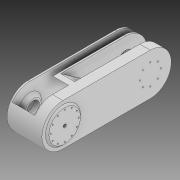
# Autodesk Inventor part: Link1
Saved by Autodesk Inventor 2020 (Build 240168000, 168)
## iProperties
Created: 2021-03-19
Part Number: Link1
Material: Generic
Document SubType Name: Modeling
Designer: DDeGo
Density: 1 g/cm^3
Appearance: Default
Author: DDeGo
Autodesk Inventor part; units mm, degrees
ref_plane "YZ Plane" through (0, 0, 0) normal (1, 0, 0) x (0, 1, 0)
ref_plane "XZ Plane" through (0, 0, 0) normal (0, 1, 0) x (-1, 0, 0)
ref_plane "XY Plane" through (0, 0, 0) normal (0, 0, 1) x (1, 0, 0)
sketch "Sketch1" plane through (0, 0, 0) normal (1, 0, 0) x (0, 1, 0)
  line L0 (0, 0) -> (0, -250) construction
  line L1 (-60, 0) -> (-60, -250)
  line L2 (60, -250) -> (60, 0)
  arc A0 (60, 0) -> (-60, 0) centre (0, 0) ccw
  arc A1 (-60, -250) -> (60, -250) centre (0, -250) ccw
  circle A2 centre (0, 0) radius 25 construction
  circle A3 centre (0, -250) radius 25
  point P0 (0, -125)
  dimension "d0" = 60
  dimension "d1" = 250
  dimension "d2" = 50
  constraints: 8 end point, 4 centre point, 4 point on circle, 4 tangent, 2 coincident, 1 equal radius, 1 midpoint, 1 parallel, 1 vertical
  measures "d0" radius of A0
  measures "d1" distance of L0.start L0.end
  measures "d2" diameter of A2
extrude "Extrusion1" add sketch "Sketch1" along normal blind 100
sketch "Sketch2" plane through (0, 60, 0) normal (0, 1, 0) x (1, 0, 0)
  line L0 (70, 185) -> (30, 185)
  line L1 (30, 185) -> (30, 315)
  line L2 (30, 315) -> (70, 315)
  line L3 (70, 315) -> (70, 185)
  line L4 (0, 250) -> (100, 250) construction
  line L5 (70, 185) -> (30, 315) construction
  line L6 (30, 185) -> (70, 315) construction
  line L7 (0, 310) -> (100, 310) construction
  line L8 (0, 250) -> (0, 310) projected
  line L9 (100, 250) -> (100, 310) projected
  point P0 (0, 0)
  point P1 (50, 250)
  dimension "d5" = 5
  dimension "d24" = 30
  dimension "d25" = 30
  constraints: 12 end point, 3 midpoint, 2 parallel, 1 horizontal, 1 perpendicular
  measures "d5" distance between parallel lines of L2 L7
  measures "d24" distance between parallel lines of L8 L1
  measures "d25" distance between parallel lines of L9 L3
extrude "Extrusion2" cut sketch "Sketch2" against normal through all
sketch "Sketch3" plane through (70, 60, -250) normal (-1, 0, 0) x (0, 0, 1)
  line L0 (0, 0) -> (65, 0) projected
  line L1 (65, 0) -> (186.3926, 0)
  line L2 (186.3926, 0) -> (65, -85)
  line L3 (65, 0) -> (65, -120) projected
  line L4 (65, -85) -> (65, 0)
  point P0 (250, -60)
  dimension "d10" = 85
  dimension "d13" = 55
  constraints: 6 end point, 1 horizontal, 1 perpendicular, 1 point on line
  measures "d10" distance of L0.end L2.end
  measures "d13" angle of L3 L2
extrude "Extrusion3" cut sketch "Sketch3" along normal up to surface (40 mm away)
sketch "Sketch4" plane through (100, 0, 0) normal (1, 0, 0) x (0, 0, -1)
  circle A0 centre (0, 0) radius 50
  dimension "d14" = 100
  constraints: 1 centre point, 1 coincident
  measures "d14" diameter of A0
extrude "Extrusion4" add sketch "Sketch4" along normal blind 5
sketch "Sketch5" plane through (105, 0, 0) normal (1, 0, 0) x (0, 0, -1)
  line L0 (0, 0) -> (40, 0) construction
  circle A0 centre (40, 0) radius 1.65
  dimension "d17" = 40
  dimension "d18" = 3.3
  constraints: 2 end point, 1 centre point, 1 coincident, 1 horizontal
  measures "d17" distance of L0.start L0.end
  measures "d18" diameter of A0
extrude "Extrusion5" cut sketch "Sketch5" against normal blind 15
pattern_circular "Circular Pattern1" count 12 over 360 about axis through (100, 0, 0) along (1, 0, 0) of "Extrusion5"
ref_plane "Work Plane1" through (5, 0, 0) normal (-1, 0, 0) x (0, 0, 1)
ref_plane "Work Plane2" through (25, 0, -250) normal (1, 0, 0) x (0, 0, -1)
sketch "Sketch7" plane through (5, 0, 0) normal (-1, 0, 0) x (0, 0, 1)
  arc A0 (0, -60) -> (0, 60) centre (0, 0) ccw projected
  line L0 (-250, 60) -> (0, 60) projected
  arc A1 (-250, 60) -> (-250, -60) centre (-250, 0) ccw projected
  line L1 (0, -60) -> (-250, -60) projected
  circle A2 centre (-250, 0) radius 25 construction
  arc A3 (0, -50) -> (50, 0) centre (0, 0) ccw
  line L2 (0, -50) -> (-250, -50)
  arc A4 (-250, 50) -> (-300, 0) centre (-250, 0) ccw construction
  line L3 (-250, 50) -> (0, 50) construction
  line L4 (50, 0) -> (50, 114.8918)
  line L5 (50, 114.8918) -> (-300, 114.8918)
  line L6 (-300, 114.8918) -> (-300, 0)
  arc A5 (50, 0) -> (0, 50) centre (0, 0) ccw construction
  arc A6 (-300, 0) -> (-250, -50) centre (-250, 0) ccw
  point P0 (-300, 33.1662)
  point P1 (50, 33.1662)
  dimension "d31" = 10
  dimension "d32" = 10
  dimension "d33" = 10
  constraints: 10 end point, 8 point on circle, 4 centre point, 2 vertical, 1 perpendicular
  measures "d31" distance between parallel lines of L1 L2
  measures "d32" radial gap between concentric circles of A0 A3
  measures "d33" radial gap between concentric circles of A1 A6
extrude "Extrusion6" cut sketch "Sketch7" against normal up to surface (20 mm away) contours L4 A3 L2 A6 L6 A1 L0 A0
sketch "Sketch8" plane through (25, 0, -300) normal (-1, 0, 0) x (0, 0, 1)
  circle A0 centre (50, 0) radius 25 projected
  line L0 (50, 60) -> (300, 60) projected
  arc A1 (50, 60) -> (0, 33.1662) centre (50, 0) ccw projected
  line L1 (0, 33.1662) -> (0, 0) projected
  arc A2 (0, 0) -> (50, -50) centre (50, 0) ccw projected
  line L2 (50, -50) -> (300, -50) projected
  arc A3 (300, -50) -> (350, 0) centre (300, 0) ccw projected
  line L3 (350, 0) -> (350, 33.1662) projected
  arc A4 (350, 33.1662) -> (300, 60) centre (300, 0) ccw projected
  line L4 (236.3926, 60) -> (115, -25) projected
  line L5 (115, -25) -> (236.3926, 60) projected
  line L6 (115, -25) -> (115, -60) projected
  line L7 (115, -25) -> (115, -60) projected
  line L8 (50, 60) -> (300, 60) projected
  line L9 (253.827, 60) -> (115, -37.2077)
  point P0 (115, -37.2077)
  point P1 (115, -50)
  dimension "d37" = 10
  constraints: 2 end point, 2 point on line, 1 parallel
  measures "d37" distance between parallel lines of L4 L9
extrude "Extrusion7" cut sketch "Sketch8" against normal up to surface (45 mm away) contours L0 A4 L3 A3 L2 L6 L9
sketch "Sketch9" plane through (0, 0, 0) normal (-1, 0, 0) x (0, 0, 1)
  circle A0 centre (0, 0) radius 17.6
  dimension "d40" = 35.2
  constraints: 1 centre point, 1 coincident
  measures "d40" diameter of A0
extrude "Extrusion8" cut sketch "Sketch9" against normal up to surface (5 mm away)
sketch "Sketch10" plane through (5, 0, 0) normal (1, 0, 0) x (0, 0, -1)
  circle A0 centre (0, 0) radius 17.6 projected
  circle A1 centre (0, 0) radius 22.6
  dimension "d43" = 5
  constraints: 1 centre point, 1 coincident
  measures "d43" radial gap between concentric circles of A1 A0
extrude "Extrusion9" add sketch "Sketch10" along normal blind 10
sketch "Sketch11" plane through (70, 0, -250) normal (-1, 0, 0) x (0, 0, 1)
  circle A0 centre (250, 0) radius 17.6 projected
  circle A1 centre (250, 0) radius 22.6
  dimension "d46" = 5
  constraints: 1 centre point, 1 coincident
  measures "d46" radial gap between concentric circles of A1 A0
extrude "Extrusion10" add sketch "Sketch11" along normal blind 10
fillet "Fillet1" radius 2 1 edges at (60, 0, -17.6)
sketch "Sketch12" plane through (105, 0, 0) normal (1, 0, 0) x (0, 0, -1)
  line L0 (4.792, 0) -> (2.396, -4.15)
  line L1 (2.396, -4.15) -> (-2.396, -4.15)
  line L2 (-2.396, -4.15) -> (-4.792, 0)
  line L3 (-4.792, 0) -> (-2.396, 4.15)
  line L4 (-2.396, 4.15) -> (2.396, 4.15)
  line L5 (2.396, 4.15) -> (4.792, 0)
  point P0 (0, 0)
  point P1 (0, 0)
  dimension "d50" = 8.3
  constraints: 12 end point, 1 coincident, 1 horizontal, 13 other
  measures "d50" distance between parallel lines of L1 L4
extrude "Extrusion11" cut sketch "Sketch12" against normal blind 6
sketch "Sketch13" plane through (99, 0, 0) normal (1, 0, 0) x (0, 0, -1)
  circle A0 centre (0, 0) radius 2.65
  dimension "d53" = 5.3
  constraints: 1 centre point, 1 coincident
  measures "d53" diameter of A0
extrude "Extrusion12" cut sketch "Sketch13" against normal blind 10
chamfer "Chamfer1" distance 10 angle 45 2 edges at (70, 0, -22.6) (5, 0, 22.6)
chamfer "Chamfer2" distance 5 angle 45 1 edges at (105, 0, 50)
sketch "Sketch14" plane through (70, 0, -250) normal (-1, 0, 0) x (0, 0, 1)
  circle A0 centre (0, 0) radius 25 projected
  circle A1 centre (0, 0) radius 47.55
  point P0 (250, 0)
  dimension "d62" = 95.1
  constraints: 1 centre point, 1 coincident
  measures "d62" diameter of A1
extrude "Extrusion13" cut sketch "Sketch14" against normal blind 10
sketch "Sketch15" plane through (80, 0, -250) normal (-1, 0, 0) x (0, 0, 1)
  circle A0 centre (0, 0) radius 25 projected
  circle A1 centre (0, 0) radius 44.55
  circle A2 centre (0, 0) radius 47.55 projected
  point P0 (250, 0)
  dimension "d65" = 3
  constraints: 1 centre point, 1 coincident
  measures "d65" radial gap between concentric circles of A2 A1
extrude "Extrusion14" cut sketch "Sketch15" against normal blind 0.5 contours A1
sketch "Sketch16" plane through (80.5, 0, -250) normal (-1, 0, 0) x (0, 0, 1)
  circle A0 centre (0, 0) radius 25 projected
  circle A1 centre (0, 0) radius 40
  point P0 (250, 0)
  dimension "d68" = 80
  constraints: 1 centre point, 1 coincident
  measures "d68" diameter of A1
extrude "Extrusion15" cut sketch "Sketch16" against normal blind 15.5
sketch "Sketch17" plane through (100, 0, 0) normal (1, 0, 0) x (0, 0, -1)
  circle A0 centre (250, 0) radius 25 construction
  circle A1 centre (250, 0) radius 30 construction
  circle A2 centre (250, 30) radius 1.6
  circle A3 centre (228.7868, 21.2132) radius 1.6
  circle A4 centre (220, 0) radius 1.6
  circle A5 centre (228.7868, -21.2132) radius 1.6
  circle A6 centre (250, -30) radius 1.6
  circle A7 centre (271.2132, -21.2132) radius 1.6
  circle A8 centre (280, 0) radius 1.6
  circle A9 centre (271.2132, 21.2132) radius 1.6
  point P0 (0, 0)
  dimension "d71" = 60
  dimension "d72" = 3.2
  dimension "d75" = 360
  constraints: 8 centre point, 2 vertical alignment, 1 coincident, 19 other
  measures "d72" diameter of A2
extrude "Extrusion16" cut sketch "Sketch17" against normal blind 15.5
sketch "Sketch18" plane through (100, 0, 0) normal (1, 0, 0) x (0, 0, -1)
  circle A0 centre (250, 0) radius 25 projected
  point P0 (0, 0)
extrude "Extrusion17" add sketch "Sketch18" against normal up to surface (4 mm away)
equation "\"d32\" = d31"
equation "\"d33\" = d31"
body "Solid1"
